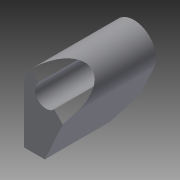
# Autodesk Inventor part: Servo Mount
Saved by Autodesk Inventor 2014 SP1 (Build 180222100, 222)
## iProperties
Created: 2014-01-26
Part Number: Servo Mount
Material: Generic
Document SubType Name: Modeling
Designer: tom
Density: 1 g/cm^3
Appearance: Default
Author: tom
Autodesk Inventor part; units mm, degrees
ref_plane "YZ Plane" through (0, 0, 0) normal (1, 0, 0) x (0, 1, 0)
ref_plane "XZ Plane" through (0, 0, 0) normal (0, 1, 0) x (-1, 0, 0)
ref_plane "XY Plane" through (0, 0, 0) normal (0, 0, 1) x (1, 0, 0)
sketch "Sketch1" plane through (0, 0, 0) normal (0, 0, 1) x (1, 0, 0)
  circle A0 centre (0, 0) radius 3.175
  circle A1 centre (0, 0) radius 6.35
  line L0 (-0.35, -16) -> (-6.35, -16)
  line L1 (-6.35, -16) -> (-6.35, 0)
  line L2 (-0.35, -16) -> (5.7723, -2.6464)
  dimension "d0" = 6.35
  dimension "d1" = 12.7
  dimension "d29" = 6
  constraints: 6 end point, 2 centre point, 2 coincident, 2 point on circle, 2 tangent
  measures "d0" diameter of A0
  measures "d1" diameter of A1
  measures "d29" distance of L0.start L0.end
extrude "Extrusion1" add sketch "Sketch1" against normal blind 25.4
body "Solid1"
